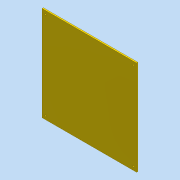
# Autodesk Inventor part: YCarriage
Saved by Autodesk Inventor 2016 (Build 200138000, 138)
## iProperties
Created: 2016-08-24
Part Number: YCarriage
Material: Dibond Yellow
Document SubType Name: Modeling
Designer: Sam
Density: 1 g/cm^3
Appearance: Generic(1)
Author: Sam
Autodesk Inventor part; units mm, degrees
ref_plane "YZ Plane" through (0, 0, 0) normal (1, 0, 0) x (0, 1, 0)
ref_plane "XZ Plane" through (0, 0, 0) normal (0, 1, 0) x (-1, 0, 0)
ref_plane "XY Plane" through (0, 0, 0) normal (0, 0, 1) x (1, 0, 0)
sketch "Sketch1" plane through (0, 0, 0) normal (0, 1, 0) x (-1, 0, 0)
  line L0 (0, 0) -> (220, 0)
  line L1 (220, 0) -> (220, -220)
  line L2 (220, -220) -> (0, -220)
  line L3 (0, -220) -> (0, 0)
  dimension "d0" = 220
  dimension "d1" = 220
  constraints: 8 end point, 2 parallel, 1 horizontal, 1 perpendicular
  measures "d0" distance of L1.end L2.end
  measures "d1" distance of L0.end L1.end
extrude "Extrusion1" add sketch "Sketch1" along normal blind 3
hole "Hole1" at (-8, 3, -8) direction (0, -1, 0) diameter 3 end through all
hole "Hole2" at (-8, 3, -212) direction (0, -1, 0) diameter 3 end through all
hole "Hole3" at (-212, 3, -8) direction (0, -1, 0) diameter 3 end through all
hole "Hole4" at (-212, 3, -212) direction (0, -1, 0) diameter 3 end through all
body "Solid1"
